Stopfen ohne loch_v2 (Autodesk Fusion 360 design; units mm, degrees)
Autodesk Fusion 360 part; units mm, degrees
cylinder "Grundkörper Zylinder1" add diameter 27 height 2.2 placed x (1, 0, 0) y (0, 0, -1) z (0, 1, 0) at (0, 0, 0)
cylinder "Grundkörper Zylinder2" add diameter 17 height 2.5 placed x (1, 0, 0) y (0, 0, -1) z (0, 1, 0) at (0, 2.2, 0)
cylinder "Grundkörper Zylinder3" add diameter 25 height 1.6 placed x (1, 0, 0) y (0, 0, -1) z (0, 1, 0) at (0, 4.7, 0)
cylinder "Grundkörper Zylinder4" add diameter 17 height 2.5 placed x (1, 0, 0) y (0, 0, -1) z (0, 1, 0) at (0, 6.3, 0)
cylinder "Grundkörper Zylinder5" add diameter 23 height 1.6 placed x (1, 0, 0) y (0, 0, -1) z (0, 1, 0) at (0, 8.8, 0)
cylinder "Grundkörper Zylinder6" add diameter 17 height 2.5 placed x (1, 0, 0) y (0, 0, -1) z (0, 1, 0) at (0, 10.4, 0)
cylinder "Grundkörper Zylinder7" add diameter 22 height 1.6 placed x (1, 0, 0) y (0, 0, -1) z (0, 1, 0) at (0, 12.9, 0)
cylinder "Grundkörper Zylinder8" add diameter 17 height 2.5 placed x (1, 0, 0) y (0, 0, -1) z (0, 1, 0) at (0, 14.5, 0)
cylinder "Grundkörper Zylinder9" add diameter 21 height 1.6 placed x (1, 0, 0) y (0, 0, -1) z (0, 1, 0) at (0, 17, 0)
cylinder "Grundkörper Zylinder10" add diameter 17 height 2.5 placed x (1, 0, 0) y (0, 0, -1) z (0, 1, 0) at (0, 18.6, 0)
cylinder "Grundkörper Zylinder11" add diameter 21 height 1.6 placed x (1, 0, 0) y (0, 0, -1) z (0, 1, 0) at (0, 21.1, 0)
cylinder "Grundkörper Zylinder12" add diameter 17 height 2.5 placed x (1, 0, 0) y (0, 0, -1) z (0, 1, 0) at (0, 22.7, 0)
cylinder "Grundkörper Zylinder13" add diameter 21 height 1.6 placed x (1, 0, 0) y (0, 0, -1) z (0, 1, 0) at (0, 25.2, 0)
cylinder "Grundkörper Zylinder14" add diameter 17 height 2.5 placed x (1, 0, 0) y (0, 0, -1) z (0, 1, 0) at (0, 26.8, 0)
cylinder "Grundkörper Zylinder15" cut diameter 12 height -84 placed x (1, 0, 0) y (0, 0, -1) z (0, 1, 0) at (0, 29.3, 0)
fillet "Abrundung1" radius 4.5 1 edges at (-7.9248, 4.7, 3.0737)
fillet "Abrundung2" radius 1 1 edges at (-7.9248, 2.2, -3.0737)
fillet "Abrundung3" radius 0.5 1 edges at (-11.6541, 4.7, -4.5202)
fillet "Abrundung4" radius 0.5 1 edges at (-11.6541, 6.3, 4.5202)
fillet "Abrundung5" radius 3 1 edges at (-7.9248, 8.8, 3.0737)
fillet "Abrundung6" radius 1 1 edges at (-7.9248, 6.3, -3.0737)
fillet "Abrundung7" radius 0.5 2 edges at (-10.7218, 8.8, -4.1586) (-10.7218, 10.4, 4.1586)
fillet "Abrundung8" radius 2.5 1 edges at (-7.9248, 12.9, 3.0737)
fillet "Abrundung9" radius 0.5 1 edges at (-7.9248, 10.4, -3.0737)
fillet "Abrundung10" radius 0.5 2 edges at (-10.2556, 12.9, -3.9778) (-10.2556, 14.5, 3.9778)
fillet "Abrundung11" radius 2 1 edges at (-7.9248, 17, 3.0737)
fillet "Abrundung12" radius 0.5 1 edges at (-7.9248, 14.5, -3.0737)
fillet "Abrundung13" radius 2 2 edges at (-7.9248, 21.1, 3.0737) (-7.9248, 25.2, 3.0737)
fillet "Abrundung14" radius 0.5 4 edges at (-7.9248, 18.6, -3.0737) (-7.9248, 22.7, -3.0737) (-7.9248, 26.8, -3.0737) (-7.9248, 29.3, 3.0737)
fillet "Abrundung15" radius 0.5 6 edges at (-9.7894, 26.8, 3.797) (-9.7894, 25.2, -3.797) (-9.7894, 22.7, 3.797) (-9.7894, 21.1, -3.797) (-9.7894, 18.6, 3.797) (-9.7894, 17, -3.797)
fillet "Abrundung16" radius 0.5 2 edges at (-12.5864, 2.2, 4.8818) (-12.5864, 0, -4.8818)
fillet "Abrundung17" radius 1.5 2 edges at (-2.1697, 29.3, 5.594) (2.1697, 0, 5.594)
